Autodesk Fusion 360 part; units mm, degrees
(part 2 of 2)
  spline S18 degree 5 poles (-7.1993, 7.4172) (-7.2053, 7.4233) (-7.2174, 7.4354) (-7.2362, 7.4528) (-7.2623, 7.4748) (-7.2964, 7.5006) (-7.3316, 7.5252) (-7.3675, 7.549) (-7.4038, 7.5725) (-7.4404, 7.5957) (-7.4772, 7.6186) (-7.5144, 7.641) (-7.5521, 7.663) (-7.5903, 7.6843) (-7.629, 7.7049) (-7.6682, 7.7251) (-7.7077, 7.7447) (-7.7476, 7.7638) (-7.7879, 7.7826) (-7.8283, 7.8011) (-7.8691, 7.8192) (-7.9101, 7.8369) (-7.9515, 7.8541) (-7.9932, 7.871) (-8.0351, 7.8874) (-8.0774, 7.9035) (-8.1199, 7.9191) (-8.1627, 7.9344) (-8.2057, 7.9494) (-8.249, 7.9639) (-8.2925, 7.9781) (-8.3363, 7.992) (-8.3802, 8.0055) (-8.4244, 8.0187) (-8.4689, 8.0314) (-8.5135, 8.0439) (-8.5584, 8.056) (-8.6035, 8.0677) (-8.6487, 8.0791) (-8.6942, 8.0902) (-8.7399, 8.1009) (-8.7858, 8.1113) (-8.8318, 8.1213) (-8.878, 8.131) (-8.9245, 8.1404) (-8.9711, 8.1495) (-9.0179, 8.1582) (-9.0648, 8.1666) (-9.1119, 8.1746) (-9.1592, 8.1824) (-9.2067, 8.1898) (-9.2543, 8.1969) (-9.302, 8.2037) (-9.35, 8.2101) (-9.398, 8.2162) (-9.4463, 8.222) (-9.4946, 8.2275) (-9.5431, 8.2327) (-9.5918, 8.2375) (-9.6406, 8.242) (-9.6895, 8.2463) (-9.7386, 8.2502) (-9.7878, 8.2537) (-9.8371, 8.257) (-9.8865, 8.26) (-9.9361, 8.2626) (-9.9858, 8.2649) (-10.0356, 8.2669) (-10.0855, 8.2686) (-10.1356, 8.27) (-10.1857, 8.2711) (-10.2259, 8.2717) (-10.2561, 8.2721) (-10.2763, 8.2722) (-10.2864, 8.2723) knots 0 0 0 0 0 0 0.01428571 0.02857143 0.04285714 0.05714286 0.07142857 0.08571429 0.1 0.11428571 0.12857143 0.14285714 0.15714286 0.17142857 0.18571429 0.2 0.21428571 0.22857143 0.24285714 0.25714286 0.27142857 0.28571429 0.3 0.31428571 0.32857143 0.34285714 0.35714286 0.37142857 0.38571429 0.4 0.41428571 0.42857143 0.44285714 0.45714286 0.47142857 0.48571429 0.5 0.51428571 0.52857143 0.54285714 0.55714286 0.57142857 0.58571429 0.6 0.61428571 0.62857143 0.64285714 0.65714286 0.67142857 0.68571429 0.7 0.71428571 0.72857143 0.74285714 0.75714286 0.77142857 0.78571429 0.8 0.81428571 0.82857143 0.84285714 0.85714286 0.87142857 0.88571429 0.9 0.91428571 0.92857143 0.94285714 0.95714286 0.97142857 0.98571429 1 1 1 1 1 1
  arc A38 (-10.2864, 8.2723) -> (-11.0461, 7.2267) centre (0, 0) ccw
  spline S19 degree 5 poles (-11.0461, 7.2267) (-11.0429, 7.2171) (-11.0365, 7.198) (-11.0269, 7.1693) (-11.0139, 7.1313) (-10.9973, 7.0839) (-10.9805, 7.0367) (-10.9635, 6.9898) (-10.9462, 6.943) (-10.9286, 6.8965) (-10.9108, 6.8502) (-10.8927, 6.8041) (-10.8744, 6.7582) (-10.8557, 6.7125) (-10.8369, 6.667) (-10.8178, 6.6218) (-10.7984, 6.5768) (-10.7787, 6.532) (-10.7588, 6.4875) (-10.7387, 6.4432) (-10.7182, 6.3991) (-10.6976, 6.3553) (-10.6766, 6.3117) (-10.6554, 6.2684) (-10.634, 6.2253) (-10.6123, 6.1824) (-10.5903, 6.1399) (-10.5681, 6.0975) (-10.5456, 6.0555) (-10.5228, 6.0137) (-10.4998, 5.9721) (-10.4765, 5.9309) (-10.453, 5.8899) (-10.4292, 5.8492) (-10.4052, 5.8088) (-10.3809, 5.7687) (-10.3563, 5.7289) (-10.3314, 5.6893) (-10.3064, 5.6501) (-10.281, 5.6111) (-10.2554, 5.5725) (-10.2295, 5.5342) (-10.2033, 5.4962) (-10.1769, 5.4586) (-10.1502, 5.4213) (-10.1232, 5.3843) (-10.096, 5.3476) (-10.0685, 5.3113) (-10.0407, 5.2754) (-10.0127, 5.2397) (-9.9844, 5.2045) (-9.9558, 5.1697) (-9.9269, 5.1353) (-9.8977, 5.1013) (-9.8682, 5.0677) (-9.8384, 5.0345) (-9.8083, 5.0017) (-9.778, 4.9693) (-9.7474, 4.9373) (-9.7166, 4.9057) (-9.6853, 4.8746) (-9.6537, 4.8442) (-9.6216, 4.8145) (-9.5891, 4.7855) (-9.5563, 4.757) (-9.5231, 4.7291) (-9.4898, 4.7014) (-9.4563, 4.6742) (-9.4225, 4.6474) (-9.3882, 4.6215) (-9.3531, 4.597) (-9.3241, 4.579) (-9.3018, 4.5665) (-9.2866, 4.5587) (-9.2789, 4.5549) knots -1 -1 -1 -1 -1 -1 -0.98571429 -0.97142857 -0.95714286 -0.94285714 -0.92857143 -0.91428571 -0.9 -0.88571429 -0.87142857 -0.85714286 -0.84285714 -0.82857143 -0.81428571 -0.8 -0.78571429 -0.77142857 -0.75714286 -0.74285714 -0.72857143 -0.71428571 -0.7 -0.68571429 -0.67142857 -0.65714286 -0.64285714 -0.62857143 -0.61428571 -0.6 -0.58571429 -0.57142857 -0.55714286 -0.54285714 -0.52857143 -0.51428571 -0.5 -0.48571429 -0.47142857 -0.45714286 -0.44285714 -0.42857143 -0.41428571 -0.4 -0.38571429 -0.37142857 -0.35714286 -0.34285714 -0.32857143 -0.31428571 -0.3 -0.28571429 -0.27142857 -0.25714286 -0.24285714 -0.22857143 -0.21428571 -0.2 -0.18571429 -0.17142857 -0.15714286 -0.14285714 -0.12857143 -0.11428571 -0.1 -0.08571429 -0.07142857 -0.05714286 -0.04285714 -0.02857143 -0.01428571 0 0 0 0 0 0
  line L19 (-9.2789, 4.5549) -> (-8.1041, 3.977)
  arc A39 (-7.7368, 3.0305) -> (-8.1041, 3.977) centre (-8.4352, 3.3041) ccw
  circle A40 centre (0, 0) radius 1.65
  circle A41 centre (0, 0) radius 3
  circle A42 centre (0, 0) radius 1.65
  line L20 (1.2445, 1.0834) -> (-1.2445, 1.0834)
  dimension "d176_1" = 6
  dimension "d177_1" = 3.3
  constraint concentric A0 A41
  constraint concentric A0 A42
  constraint coincident A42 L20.end
  constraint coincident A42 L20.start
  constraint horizontal L20
  measures "d176_1" diameter of A41
  measures "d177_1" diameter of A42
extrude "Extrude3" add sketch "gear motor detailed cut" against normal blind 4 contours A40 A42 L20 picked at (-0.2966, 1.1854) in component "gear motor (1)"
extrude "Extrude4" add sketch "gear motor detailed cut" along normal blind 6 contours A40 A42 L20 | A41 picked at (-0.2966, 1.1854) in component "gear motor (1)"
component "gear motor (1)" placed x (1, 0, 0) y (0, 1, 0) z (0, 0, 1) at (0, 0, 0)
equation "distanceOne_1 = 4.00 mm"
equation "taperAngle1_1 = 0.0 deg"
equation "Radius_1 = 0.75 mm"
equation "countU_1 = 10"
named bodies: "gear motor"
